Autodesk Fusion 360 part; units mm, degrees
(part 3 of 3)
sketch "connector_2 profile" plane through (0, 0, -325) normal (0, 0, 1) x (1, 0, 0) in component "rear_interfaces | Rear connections | revision 0.3"
  line L0 (-34, 161.5) -> (-6, 161.5)
  line L1 (-6, 161.5) -> (-6, 178.5)
  line L2 (-6, 178.5) -> (-34, 178.5)
  line L3 (-34, 178.5) -> (-34, 161.5)
extrude "connector_2 native extrusion" add sketch "connector_2 profile" along normal blind 6 separate body makes body 321 in component "rear_interfaces | Rear connections | revision 0.3"
ref_plane "WorkPlane4" through (0, 0, -325) normal (0, 0, 1) x (1, 0, 0) in component "rear_interfaces | Rear connections | revision 0.3"
sketch "connector_3 profile" plane through (0, 0, -325) normal (0, 0, 1) x (1, 0, 0) in component "rear_interfaces | Rear connections | revision 0.3"
  line L0 (26, 161.5) -> (54, 161.5)
  line L1 (54, 161.5) -> (54, 178.5)
  line L2 (54, 178.5) -> (26, 178.5)
  line L3 (26, 178.5) -> (26, 161.5)
extrude "connector_3 native extrusion" add sketch "connector_3 profile" along normal blind 6 separate body makes body 322 in component "rear_interfaces | Rear connections | revision 0.3"
ref_plane "WorkPlane5" through (0, 0, -325) normal (0, 0, 1) x (1, 0, 0) in component "rear_interfaces | Rear connections | revision 0.3"
sketch "connector_4 profile" plane through (0, 0, -325) normal (0, 0, 1) x (1, 0, 0) in component "rear_interfaces | Rear connections | revision 0.3"
  line L0 (86, 161.5) -> (114, 161.5)
  line L1 (114, 161.5) -> (114, 178.5)
  line L2 (114, 178.5) -> (86, 178.5)
  line L3 (86, 178.5) -> (86, 161.5)
extrude "connector_4 native extrusion" add sketch "connector_4 profile" along normal blind 6 separate body makes body 323 in component "rear_interfaces | Rear connections | revision 0.3"
ref_plane "WorkPlane6" through (0, 0, -323.5) normal (0, 0, 1) x (1, 0, 0) in component "rear_interfaces | Rear connections | revision 0.3"
sketch "vent_slot profile" plane through (0, 0, -323.5) normal (0, 0, 1) x (1, 0, 0) in component "rear_interfaces | Rear connections | revision 0.3"
  line L0 (120, 253.5) -> (240, 253.5)
  line L1 (240, 253.5) -> (240, 256.5)
  line L2 (240, 256.5) -> (120, 256.5)
  line L3 (120, 256.5) -> (120, 253.5)
  line L4 (120, 262.5) -> (240, 262.5)
  line L5 (240, 262.5) -> (240, 265.5)
  line L6 (240, 265.5) -> (120, 265.5)
  line L7 (120, 265.5) -> (120, 262.5)
  line L8 (120, 271.5) -> (240, 271.5)
  line L9 (240, 271.5) -> (240, 274.5)
  line L10 (240, 274.5) -> (120, 274.5)
  line L11 (120, 274.5) -> (120, 271.5)
  line L12 (120, 280.5) -> (240, 280.5)
  line L13 (240, 280.5) -> (240, 283.5)
  line L14 (240, 283.5) -> (120, 283.5)
  line L15 (120, 283.5) -> (120, 280.5)
  line L16 (120, 289.5) -> (240, 289.5)
  line L17 (240, 289.5) -> (240, 292.5)
  line L18 (240, 292.5) -> (120, 292.5)
  line L19 (120, 292.5) -> (120, 289.5)
  line L20 (120, 298.5) -> (240, 298.5)
  line L21 (240, 298.5) -> (240, 301.5)
  line L22 (240, 301.5) -> (120, 301.5)
  line L23 (120, 301.5) -> (120, 298.5)
  line L24 (120, 307.5) -> (240, 307.5)
  line L25 (240, 307.5) -> (240, 310.5)
  line L26 (240, 310.5) -> (120, 310.5)
  line L27 (120, 310.5) -> (120, 307.5)
  line L28 (120, 316.5) -> (240, 316.5)
  line L29 (240, 316.5) -> (240, 319.5)
  line L30 (240, 319.5) -> (120, 319.5)
  line L31 (120, 319.5) -> (120, 316.5)
  line L32 (120, 325.5) -> (240, 325.5)
  line L33 (240, 325.5) -> (240, 328.5)
  line L34 (240, 328.5) -> (120, 328.5)
  line L35 (120, 328.5) -> (120, 325.5)
  line L36 (120, 334.5) -> (240, 334.5)
  line L37 (240, 334.5) -> (240, 337.5)
  line L38 (240, 337.5) -> (120, 337.5)
  line L39 (120, 337.5) -> (120, 334.5)
  line L40 (120, 343.5) -> (240, 343.5)
  line L41 (240, 343.5) -> (240, 346.5)
  line L42 (240, 346.5) -> (120, 346.5)
  line L43 (120, 346.5) -> (120, 343.5)
  line L44 (120, 352.5) -> (240, 352.5)
  line L45 (240, 352.5) -> (240, 355.5)
  line L46 (240, 355.5) -> (120, 355.5)
  line L47 (120, 355.5) -> (120, 352.5)
extrude "vent_slot native extrusion" add sketch "vent_slot profile" along normal blind 3 separate body makes body 324 at (200, 346.5, -322.5) makes body 325 at (200, 326.5, -323.5) makes body 326 at (200, 310.5, -322.5) makes body 327 at (200, 301.5, -322.5) makes body 328 at (200, 283.5, -322.5) makes body 329 at (200, 265.5, -322.5) makes body 330 at (200, 274.5, -322.5) makes body 331 at (200, 292.5, -322.5) makes body 332 at (200, 256.5, -322.5) makes body 333 at (200, 319.5, -322.5) makes body 334 at (200, 337.5, -322.5) makes body 335 at (200, 355.5, -322.5) in component "rear_interfaces | Rear connections | revision 0.3"
ref_plane "WorkPlane1" through (0, 0, 7.5) normal (0, 0, 1) x (1, 0, 0) in component "monitor | Adjacent monitor - 650 mm wide | revision 0.3"
sketch "monitor_housing profile" plane through (0, 0, 7.5) normal (0, 0, 1) x (1, 0, 0) in component "monitor | Adjacent monitor - 650 mm wide | revision 0.3"
  line L0 (445, 170) -> (1095, 170)
  line L1 (1095, 170) -> (1095, 580)
  line L2 (1095, 580) -> (445, 580)
  line L3 (445, 580) -> (445, 170)
extrude "monitor_housing native extrusion" add sketch "monitor_housing profile" along normal blind 35 separate body makes body 336 in component "monitor | Adjacent monitor - 650 mm wide | revision 0.3"
ref_plane "WorkPlane2" through (0, 0, 42.5) normal (0, 0, 1) x (1, 0, 0) in component "monitor | Adjacent monitor - 650 mm wide | revision 0.3"
sketch "monitor_screen profile" plane through (0, 0, 42.5) normal (0, 0, 1) x (1, 0, 0) in component "monitor | Adjacent monitor - 650 mm wide | revision 0.3"
  line L0 (459, 188) -> (1081, 188)
  line L1 (1081, 188) -> (1081, 568)
  line L2 (1081, 568) -> (459, 568)
  line L3 (459, 568) -> (459, 188)
extrude "monitor_screen native extrusion" add sketch "monitor_screen profile" along normal blind 2 separate body makes body 337 in component "monitor | Adjacent monitor - 650 mm wide | revision 0.3"
ref_plane "WorkPlane3" through (0, 0, -8) normal (0, 0, 1) x (1, 0, 0) in component "monitor | Adjacent monitor - 650 mm wide | revision 0.3"
sketch "monitor_stem profile" plane through (0, 0, -8) normal (0, 0, 1) x (1, 0, 0) in component "monitor | Adjacent monitor - 650 mm wide | revision 0.3"
  line L0 (749, 14) -> (791, 14)
  line L1 (791, 14) -> (791, 170)
  line L2 (791, 170) -> (749, 170)
  line L3 (749, 170) -> (749, 14)
extrude "monitor_stem native extrusion" add sketch "monitor_stem profile" along normal blind 40 separate body makes body 338 in component "monitor | Adjacent monitor - 650 mm wide | revision 0.3"
ref_plane "WorkPlane4" through (0, 0, -65) normal (0, 0, 1) x (1, 0, 0) in component "monitor | Adjacent monitor - 650 mm wide | revision 0.3"
sketch "monitor_base profile" plane through (0, 0, -65) normal (0, 0, 1) x (1, 0, 0) in component "monitor | Adjacent monitor - 650 mm wide | revision 0.3"
  line L0 (627.5, 0) -> (912.5, 0)
  line L1 (912.5, 0) -> (912.5, 14)
  line L2 (912.5, 14) -> (627.5, 14)
  line L3 (627.5, 14) -> (627.5, 0)
extrude "monitor_base native extrusion" add sketch "monitor_base profile" along normal blind 180 separate body makes body 339 in component "monitor | Adjacent monitor - 650 mm wide | revision 0.3"
ref_plane "WorkPlane5" through (0, 0, 325) normal (0, 0, 1) x (1, 0, 0) in component "base | Base and nominal envelope | revision 0.3"
sketch "Sketch5" plane through (0, 0, 325) normal (0, 0, 1) x (1, 0, 0) in component "base | Base and nominal envelope | revision 0.3"
  line L0 (-325, 42) -> (325, 42)
  line L1 (325, 42) -> (325, 98)
  line L2 (325, 98) -> (-325, 98)
  line L3 (-325, 98) -> (-325, 42)
extrude "lower_front_fascia" add sketch "Sketch5" along normal blind 26 separate body makes body 340 in component "base | Base and nominal envelope | revision 0.3"
ref_plane "WorkPlane6" through (0, 0, 325) normal (0, 0, 1) x (1, 0, 0) in component "base | Base and nominal envelope | revision 0.3"
sketch "Sketch6" plane through (0, 0, 325) normal (0, 0, 1) x (1, 0, 0) in component "base | Base and nominal envelope | revision 0.3"
  line L0 (-325, 14) -> (325, 14)
  line L1 (325, 14) -> (325, 42)
  line L2 (325, 42) -> (-325, 42)
  line L3 (-325, 42) -> (-325, 14)
extrude "bottom_front_trim" add sketch "Sketch6" along normal blind 28 separate body makes body 341 in component "base | Base and nominal envelope | revision 0.3"
ref_plane "WorkPlane1" through (0, 0, 332.5) normal (0, 0, 1) x (1, 0, 0) in component "cassette_door | Overlapping sliding door | revision 0.4"
sketch "Door perimeter - 2 mm frame overlap, 1 mm bottom reveal" plane through (0, 0, 332.5) normal (0, 0, 1) x (1, 0, 0) in component "cassette_door | Overlapping sliding door | revision 0.4"
  line L0 (60, 120) -> (313, 120)
  line L1 (313, 120) -> (313, 610)
  arc A0 (313, 610) -> (235, 688) centre (235, 610) ccw
  line L2 (235, 688) -> (60, 688)
  line L3 (60, 688) -> (60, 508)
  line L4 (60, 508) -> (26, 474)
  line L5 (26, 474) -> (26, 366)
  line L6 (26, 366) -> (60, 332)
  line L7 (60, 332) -> (60, 120)
extrude "sliding_cover_notched native extrusion" add sketch "Door perimeter - 2 mm frame overlap, 1 mm bottom reveal" along normal blind 13 separate body makes body 342 in component "cassette_door | Overlapping sliding door | revision 0.4"
ref_plane "WorkPlane2" through (0, 0, 346) normal (0, 0, 1) x (1, 0, 0) in component "cassette_door | Overlapping sliding door | revision 0.4"
sketch "Sketch2" plane through (0, 0, 346) normal (0, 0, 1) x (1, 0, 0) in component "cassette_door | Overlapping sliding door | revision 0.4"
  line L0 (276.5, 336) -> (291.5, 336)
  line L1 (291.5, 336) -> (291.5, 464)
  line L2 (291.5, 464) -> (276.5, 464)
  line L3 (276.5, 464) -> (276.5, 336)
extrude "handle" add sketch "Sketch2" along normal blind 12 separate body makes body 343 in component "cassette_door | Overlapping sliding door | revision 0.4"
component "cassette_bays | Three vertical cassette bays | DEPTH PROVISIONAL" placed x (1, 0, 0) y (0, 1, 0) z (0, 0, 1) at (0, 0, 0)
component "cassette_0 | Bottom cassette | DEPTH PROVISIONAL" placed x (1, 0, 0) y (0, 1, 0) z (0, 0, 1) at (0, 0, 0)
component "cassette_1 | Middle cassette | DEPTH PROVISIONAL" placed x (1, 0, 0) y (0, 1, 0) z (0, 0, 1) at (0, 0, 0)
component "cassette_2 | Top cassette | DEPTH PROVISIONAL" placed x (1, 0, 0) y (0, 1, 0) z (0, 0, 1) at (0, 0, 0)
component "imaging_stage | Imaging stage (schematic)" placed x (1, 0, 0) y (0, 1, 0) z (0, 0, 1) at (0, 0, 0)
component "optics | Objective and condenser (schematic)" placed x (1, 0, 0) y (0, 1, 0) z (0, 0, 1) at (0, 0, 0)
component "calibration_storage | Calibration-slide compartment" placed x (1, 0, 0) y (0, 1, 0) z (0, 0, 1) at (0, 0, 0)
component "base | Base and nominal envelope | revision 0.3" placed x (1, 0, 0) y (0, 1, 0) z (0, 0, 1) at (0, 0, 0)
component "enclosure | Enclosure - revised silhouette | revision 0.3" placed x (1, 0, 0) y (0, 1, 0) z (0, 0, 1) at (0, 0, 0)
component "front_controls | Front control strip | revision 0.3" placed x (1, 0, 0) y (0, 1, 0) z (0, 0, 1) at (0, 0, 0)
component "rear_interfaces | Rear connections | revision 0.3" placed x (1, 0, 0) y (0, 1, 0) z (0, 0, 1) at (0, 0, 0)
component "monitor | Adjacent monitor - 650 mm wide | revision 0.3" placed x (1, 0, 0) y (0, 1, 0) z (0, 0, 1) at (0, 0, 0)
component "cassette_door | Overlapping sliding door | revision 0.4" placed x (1, 0, 0) y (0, 1, 0) z (0, 0, 1) at (0, 0, 0)
equation "BodyWidth = 650 mm" comment "Manual PDF 19-20; excludes protrusions"
equation "BodyDepth = 650 mm" comment "Manual PDF 19-21; excludes protrusions"
equation "BodyHeight = 700 mm" comment "Manual PDF 20; exterior envelope"
equation "MEASURE_REQUIRED_DoorInnerZ = 332.5 mm" comment "Provisional door datum, not OEM measurement"
equation "MEASURE_REQUIRED_DoorToHolderFront = 500 mm" comment "PROVISIONAL layout gap, NOT specified in manual. Closed door INNER face to holder frame FRONT"
equation "MEASURE_REQUIRED_HolderHalfDepth = 54 mm" comment "Provisional holder frame half-depth"
equation "CassetteCentreZ = MEASURE_REQUIRED_DoorInnerZ - MEASURE_REQUIRED_DoorToHolderFront - MEASURE_REQUIRED_HolderHalfDepth" comment "Dependent rear-cassette depth"
equation "MEASURE_REQUIRED_DoorTravel = 225 mm" comment "Direction documented: left to open; travel unmeasured"
equation "MEASURE_REQUIRED_CassetteWidth = 80 mm" comment "Unmeasured"
equation "MEASURE_REQUIRED_CassetteDepth = 96 mm" comment "Unmeasured"
equation "MEASURE_REQUIRED_CassetteHeight = 126 mm" comment "Unmeasured"
equation "MEASURE_REQUIRED_SlotPitch = 10.5 mm" comment "Unmeasured"
equation "d61 = CassetteCentreZ + -58.5 mm"
equation "d65 = CassetteCentreZ + -54.0 mm"
equation "d69 = CassetteCentreZ + -54.0 mm"
equation "d73 = CassetteCentreZ + 56.0 mm"
equation "d77 = CassetteCentreZ + 56.0 mm"
equation "d81 = CassetteCentreZ + 56.0 mm"
equation "d85 = CassetteCentreZ + -48.0 mm"
equation "d89 = CassetteCentreZ + -48.0 mm"
equation "d93 = CassetteCentreZ + -48.0 mm"
equation "d97 = CassetteCentreZ + 44.0 mm"
equation "d101 = CassetteCentreZ + -12.5 mm"
equation "d105 = CassetteCentreZ + -48.0 mm"
equation "d109 = CassetteCentreZ + -38.0 mm"
equation "d113 = CassetteCentreZ + -41.5 mm"
equation "d117 = CassetteCentreZ + -48.0 mm"
equation "d121 = CassetteCentreZ + -48.0 mm"
equation "d125 = CassetteCentreZ + -48.0 mm"
equation "d129 = CassetteCentreZ + 44.0 mm"
equation "d133 = CassetteCentreZ + -12.5 mm"
equation "d137 = CassetteCentreZ + -48.0 mm"
equation "d141 = CassetteCentreZ + -38.0 mm"
equation "d145 = CassetteCentreZ + -41.5 mm"
equation "d149 = CassetteCentreZ + -48.0 mm"
equation "d153 = CassetteCentreZ + -48.0 mm"
equation "d157 = CassetteCentreZ + -48.0 mm"
equation "d161 = CassetteCentreZ + 44.0 mm"
equation "d165 = CassetteCentreZ + -12.5 mm"
equation "d169 = CassetteCentreZ + -48.0 mm"
equation "d173 = CassetteCentreZ + -38.0 mm"
equation "d177 = CassetteCentreZ + -41.5 mm"
equation "OverallWidth = 685 mm" comment "Brochure overall scanner width including protrusions"
equation "OverallDepth = 683 mm" comment "Original S60 brochure overall scanner depth"
equation "MonitorWidth = 650 mm" comment "Visiopharm brochure page 2 monitor width; other monitor dimensions estimated"
equation "PHOTO_ESTIMATE_CornerRadius = 90 mm" comment "Upper-right enclosure corner; appearance estimate, not OEM dimension"
named bodies: "bay_back_1", "side_frame_1", "side_frame_2", "cross_frame_1", "cross_frame_2", "cross_frame_3", "cross_frame_4", "seat_led_0_1", "seat_led_1_1", "seat_led_2_1", "rack_base_1", "rack_top_1", "outer_guide_1", "outer_guide_2", "rear_rib_PHOTO_ESTIMATE_1", "rear_rib_PHOTO_ESTIMATE_2", "rear_rib_PHOTO_ESTIMATE_3", "magnetic_base_1", "center_divider_1", "slide_glass_1", "slide_glass_2", "slide_glass_3", "slide_glass_4", "slide_glass_5", "slide_glass_6", "slide_glass_7", "slide_glass_8", "slide_glass_9", "slide_glass_10", "slide_glass_11", "slide_glass_12", "slide_glass_13", "slide_glass_14", "slide_glass_15", "slide_glass_16", "slide_glass_17", "slide_glass_18", "slide_glass_19", "slide_glass_20", "slot_guide_1", "slot_guide_2", "slot_guide_3", "slot_guide_4", "slot_guide_5", "slot_guide_6", "slot_guide_7", "slot_guide_8", "slot_guide_9", "slot_guide_10", "slot_guide_11", "slot_guide_12", "slot_guide_13", "slot_guide_14", "slot_guide_15", "slot_guide_16", "slot_guide_17", "slot_guide_18", "slot_guide_19", "slot_guide_20", "slot_guide_21", "slot_guide_22", "slot_guide_23", "slot_guide_24", "slot_guide_25", "slot_guide_26", "slot_guide_27", "slot_guide_28", "slot_guide_29", "slot_guide_30", "slot_guide_31", "slot_guide_32", "slot_guide_33", "slot_guide_34", "slot_guide_35", "slot_guide_36", "slot_guide_37", "slot_guide_38", "slot_guide_39", "slot_guide_40", "stage_base_1", "stage_plate_1", "glass_seat_1", "objective_20x_NA075_1", "interchangeable_condenser_1", "Calibration slide 1", "Calibration slide 2", "Calibration slide 3", "Calibration slide 4", "base_plate_1", "lower_body_band_1", "foot_1", "foot_2", "foot_1 (1)", "foot_2 (1)", "rounded_casing_1", "rear_panel_1", "front_perimeter_1", "fixed_front_notched_1", "front_sill_1", "left_service_hinge_1", "left_service_hinge_2", "right_service_latch_1", "right_service_latch_2", "right_service_panel_1", "right_service_handle_1", "side_vent_1", "side_vent_2", "side_vent_3", "side_vent_4", "side_vent_5", "side_vent_1 (1)", "side_vent_2 (1)", "side_vent_3 (1)", "side_vent_4 (1)", "side_vent_5 (1)", "side_vent_1 (2)", "side_vent_2 (2)", "side_vent_3 (2)", "side_vent_4 (2)", "side_vent_5 (2)", "side_vent_1 (3)", "side_vent_2 (3)", "side_vent_3 (3)", "side_vent_4 (3)", "side_vent_5 (3)", "side_vent_1 (4)", "side_vent_2 (4)", "side_vent_3 (4)", "side_vent_4 (4)", "side_vent_5 (4)", "side_vent_1 (5)", "side_vent_2 (5)", "side_vent_3 (5)", "side_vent_4 (5)", "side_vent_5 (5)", "side_vent_1 (6)", "side_vent_2 (6)", "side_vent_3 (6)", "side_vent_4 (6)", "side_vent_5 (6)", "side_vent_1 (7)", "side_vent_2 (7)", "side_vent_3 (7)", "side_vent_4 (7)", "side_vent_5 (7)", "side_vent_1 (8)", "side_vent_2 (8)", "side_vent_3 (8)", "side_vent_4 (8)", "side_vent_5 (8)", "side_vent_1 (9)", "side_vent_2 (9)", "side_vent_3 (9)", "side_vent_4 (9)", "side_vent_5 (9)", "side_vent_1 (10)", "side_vent_2 (10)", "side_vent_3 (10)", "side_vent_4 (10)", "side_vent_5 (10)", "side_vent_1 (11)", "side_vent_2 (11)", "side_vent_3 (11)", "side_vent_4 (11)", "side_vent_5 (11)", "side_vent_1 (12)", "side_vent_2 (12)", "side_vent_3 (12)", "side_vent_4 (12)", "side_vent_5 (12)", "side_vent_1 (13)", "side_vent_2 (13)", "side_vent_3 (13)", "side_vent_4 (13)", "side_vent_5 (13)", "control_recess_1", "led_0_1", "led_1_1", "led_2_1", "power_switch_1", "connector_0_1", "connector_1_1", "connector_2_1", "connector_3_1", "connector_4_1", "vent_slot_1", "vent_slot_2", "vent_slot_3", "vent_slot_4", "vent_slot_5", "vent_slot_6", "vent_slot_7", "vent_slot_8", "vent_slot_9", "vent_slot_10", "vent_slot_11", "vent_slot_12", "monitor_housing_1", "monitor_screen_1", "monitor_stem_1", "monitor_base_1", "lower_front_fascia", "bottom_front_trim", "sliding_cover_notched", "handle"
